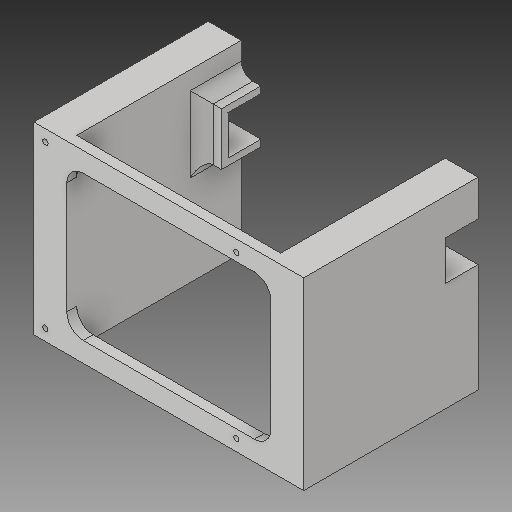
# Autodesk Inventor part: baseRaspberry
Saved by Autodesk Inventor 2018 (Build 220112000, 112)
## iProperties
Created: 2018-02-26
Part Number: baseRaspberry
Material: Genérico
Document SubType Name: Modeling
Designer: ivanb
Density: 1 g/cm^3
Appearance: Valor por defecto
Author: ivanb
Autodesk Inventor part; units mm, degrees
ref_plane "YZ Plane" through (0, 0, 0) normal (1, 0, 0) x (0, 1, 0)
ref_plane "XZ Plane" through (0, 0, 0) normal (0, 1, 0) x (-1, 0, 0)
ref_plane "XY Plane" through (0, 0, 0) normal (0, 0, 1) x (1, 0, 0)
ref_plane "Plano de trabajo1" through (-77.1004, 28.9483, 0) normal (0, 0, -1) x (-1, 0, 0)
sketch "Boceto1" plane through (-77.1004, 28.9483, 0) normal (0, 0, -1) x (-1, 0, 0)
  line L0 (82, -56) -> (-3, -56)
  line L1 (-3, -56) -> (-3, 0)
  line L2 (-3, 0) -> (82, 0)
  line L3 (82, 0) -> (82, -56)
  point P0 (-77.1004, -28.9483)
  constraints: 8 end point, 2 parallel, 1 horizontal, 1 perpendicular
extrude "Extrusión1" add sketch "Boceto1" along normal blind 20
ref_plane "Plano de trabajo3" through (-77.1004, 28.9483, 0) normal (0, 0, 1) x (1, 0, 0)
sketch "Boceto2" plane through (-77.1004, 28.9483, 0) normal (0, 0, 1) x (1, 0, 0)
  circle A0 centre (-78.5, -3.5) radius 1.375 projected
  circle A1 centre (-78.5, -3.5) radius 1.125
  circle A2 centre (-20.5, -3.5) radius 1.375 projected
  circle A3 centre (-20.5, -3.5) radius 1.125
  circle A4 centre (-20.5, -52.5) radius 1.375 projected
  circle A5 centre (-20.5, -52.5) radius 1.125
  circle A6 centre (-78.5, -52.5) radius 1.375 projected
  circle A7 centre (-78.5, -52.5) radius 1.125
  line L0 (-91.1268, 5.8368) -> (25.5851, 5.8368)
  line L1 (25.5851, 5.8368) -> (25.5851, -70.6743)
  line L2 (25.5851, -70.6743) -> (-91.1268, -70.6743)
  line L3 (-91.1268, -70.6743) -> (-91.1268, 5.8368)
  point P0 (77.1004, -28.9483)
  dimension "d3" = 2.25
  dimension "d4" = 2.25
  dimension "d5" = 2.25
  dimension "d6" = 2.25
  constraints: 8 end point, 4 centre point, 4 coincident, 2 parallel, 1 horizontal, 1 perpendicular
  measures "d3" diameter of A1
  measures "d4" diameter of A3
  measures "d5" diameter of A5
  measures "d6" diameter of A7
extrude "Extrusión2" cut sketch "Boceto2" against normal blind 10 contours L0 L1 L2 L3
ref_plane "Plano de trabajo2" through (-77.1004, 28.9483, -20) normal (0, 0, -1) x (-1, 0, 0)
sketch "Boceto8" plane through (-77.1004, 28.9483, -20) normal (0, 0, -1) x (-1, 0, 0)
  circle A0 centre (77, -31) radius 1.25
  circle A1 centre (77, -3) radius 1.25
  line L0 (-3, -56) -> (82, -56) projected
  circle A2 centre (5, -31) radius 1.25
  circle A3 centre (5, -3) radius 1.25
  line L1 (82, -56) -> (82, 0) projected
  line L2 (82, -56) -> (72, -56)
  line L3 (72, -56) -> (72, 0)
  line L4 (72, 0) -> (82, 0)
  line L5 (82, 0) -> (82, -56)
  line L6 (10.1328, -56) -> (0.1328, -56)
  line L7 (5, -31) -> (5, -3)
  line L8 (0, -52.0097) -> (0, -25.6767)
  line L9 (79, -56) -> (0, -56) projected
  line L10 (0, -56) -> (10, -56)
  line L11 (10, -56) -> (10, 0)
  line L12 (10, 0) -> (0, 0)
  line L13 (0, 0) -> (0, -56)
  line L14 (82, 0) -> (-3, 0) projected
  point P0 (-77.1004, -28.9483)
  dimension "d31" = 2.5
  dimension "d32" = 2.5
  dimension "d33" = 28
  dimension "d35" = 2.5
  dimension "d36" = 72
  dimension "d37" = 2.5
  dimension "d38" = 5
  dimension "d39" = 72
  dimension "d40" = 5
  dimension "d41" = 28
  dimension "d43" = 10
  dimension "d45" = 5
  dimension "d46" = 10
  dimension "d92" = 0
  dimension "d175" = 3
  dimension "d176" = 3
  constraints: 22 end point, 4 centre point, 4 parallel, 3 horizontal, 2 perpendicular, 1 point on line, 1 vertical
  measures "d31" diameter of A0
  measures "d32" diameter of A1
  measures "d33" distance of A1.centre A0.centre
  measures "d35" diameter of A2
  measures "d36" distance of L7.start A0.centre
  measures "d37" diameter of A3
  measures "d38" distance from line of L1 A0.centre
  measures "d39" distance of L7.end A1.centre
  measures "d40" distance from line of L1 A1.centre
  measures "d41" distance of L7.end L7.start
  measures "d43" distance of L3.end L4.end
  measures "d45" distance from line of L7.start L8
  measures "d46" distance of L12.end L11.end
  measures "d92" distance between parallel lines of L14 L12
  measures "d175" distance from line of L14 L7.end
  measures "d176" distance from line of L14 A1.centre
extrude "Extrusión8" add sketch "Boceto8" along normal blind 30 contours L13 L8 L12 L11 L0 | L3 L4 L1 L0
ref_plane "Plano de trabajo6" through (-159.1004, -27.0517, -10) normal (-1, 0, 0) x (0, 0, 1)
sketch "Boceto9" plane through (-159.1004, -27.0517, -10) normal (-1, 0, 0) x (0, 0, 1)
  line L0 (-30, 33) -> (-40, 33)
  line L1 (-40, 33) -> (-40, 45)
  line L2 (-40, 45) -> (-30, 45)
  line L3 (-30, 45) -> (-30, 33)
  line L4 (0, 0) -> (-40, 0) projected
  line L5 (-40, 0) -> (-40, 56) projected
  line L6 (0, 56) -> (-40, 56) projected
  point P0 (10, 27.0517)
  dimension "d49" = 10
  dimension "d50" = 12
  dimension "d52" = 0
  dimension "d82" = 11
  constraints: 8 end point, 2 parallel, 1 horizontal, 1 perpendicular
  measures "d49" distance of L1.end L2.end
  measures "d50" distance of L0.end L1.end
  measures "d52" distance between parallel lines of L5 L1
  measures "d82" distance between parallel lines of L6 L2
extrude "Extrusión9" cut sketch "Boceto9" against normal blind 100
ref_plane "Plano de trabajo5" through (-149.1004, -27.0517, -20) normal (1, 0, 0) x (0, 0, -1)
sketch "Boceto10" plane through (-149.1004, -27.0517, -20) normal (1, 0, 0) x (0, 0, -1)
  line L0 (18, 31) -> (30, 31)
  line L1 (30, 31) -> (30, 47)
  line L2 (30, 47) -> (18, 47)
  line L3 (18, 47) -> (18, 31)
  line L4 (-10, 56) -> (30, 56) projected
  line L5 (30, 33) -> (30, 0) projected
  line L6 (20, 33) -> (20, 45) projected
  line L7 (30, 33) -> (20, 33)
  line L8 (20, 33) -> (20, 45)
  line L9 (20, 45) -> (30, 45) projected
  line L10 (20, 45) -> (30, 45)
  point P0 (-20, 27.0517)
  dimension "d59" = 12
  dimension "d60" = 16
  dimension "d133" = 2
  constraints: 14 end point, 4 equal length, 2 perpendicular, 1 horizontal
  measures "d59" distance of L0.start L0.end
  measures "d60" distance of L0.end L1.end
  measures "d133" distance between parallel lines of L9 L2
extrude "Extrusión10" add sketch "Boceto10" along normal blind 6 contours L3 L2 L1 L9 L6 L7 L0
sketch "Boceto11" plane through (-77.1004, -27.0517, -20) normal (1, 0, 0) x (0, 0, -1)
  line L0 (30, 45) -> (30, 76)
  line L1 (18, 31) -> (30, 31)
  line L2 (30, 31) -> (30, 47)
  line L3 (30, 47) -> (18, 47)
  line L4 (18, 47) -> (18, 31)
  line L5 (30, 33) -> (20, 33)
  line L6 (20, 33) -> (30, 33)
  line L7 (30, 33) -> (20, 33)
  line L8 (20, 33) -> (20, 45)
  line L9 (20, 33) -> (20, 45)
  line L10 (30, 45) -> (20, 45)
  line L11 (20, 45) -> (30, 45)
  line L12 (20, 45) -> (30, 45) projected
  point P0 (-20, 27.0517)
  point P1 (-20, 27.0517)
  dimension "d64" = 12
  dimension "d65" = 16
  dimension "d66" = 2
  dimension "d88" = 0
  dimension "d89" = 2
  dimension "d177" = 10
  constraints: 24 end point, 3 equal length, 3 perpendicular, 1 horizontal, 1 point on line
  measures "d64" distance of L1.start L1.end
  measures "d65" distance of L1.end L2.end
  measures "d66" distance between parallel lines of L1 L5
  measures "d88" distance between parallel lines of L12 L10
  measures "d89" distance between parallel lines of L3 L10
  measures "d177" distance of L0.start L8.end
extrude "Extrusión11" add sketch "Boceto11" against normal blind 16 contours L10 L8 L5 L2 L1 L4 L3 L0
ref_plane "Plano de trabajo4" through (-159.1004, -27.0517, -10) normal (0, -1, 0) x (1, 0, 0)
sketch "Boceto12" plane through (-159.1004, -27.0517, -10) normal (0, -1, 0) x (1, 0, 0)
  line L0 (0, 0) -> (0, -40) projected
  line L1 (0, -7) -> (97.2238, -7)
  line L2 (97.2238, -7) -> (97.2238, 2.4478)
  line L3 (97.2238, 2.4478) -> (0, 2.4478)
  line L4 (0, 2.4478) -> (0, -7)
  line L5 (72, -10) -> (10, -10) projected
  point P0 (159.1004, 10)
  dimension "d69" = 3
  constraints: 8 end point, 2 parallel, 1 horizontal, 1 perpendicular, 1 point on line
  measures "d69" distance between parallel lines of L1 L5
extrude "Extrusión12" cut sketch "Boceto12" against normal blind 60
sketch "Boceto13" plane through (-155.6004, 25.4483, 0) normal (0, 0, 1) x (1, 0, 0)
  line L0 (90.0679, 13.1573) -> (-12.4886, 13.1573)
  line L1 (-12.4886, 13.1573) -> (-12.4886, -64.4116)
  line L2 (-12.4886, -64.4116) -> (90.0679, -64.4116)
  line L3 (90.0679, -64.4116) -> (90.0679, 13.1573)
  point P0 (155.6004, -25.4483)
  constraints: 8 end point, 2 parallel, 1 horizontal, 1 perpendicular
extrude "Extrusión13" cut sketch "Boceto13" against normal blind 10
ref_plane "Plano de trabajo8" through (-159.1004, -27.0517, -17) normal (0, 0, 1) x (1, 0, 0)
sketch "Boceto14" plane through (-159.1004, -27.0517, -17) normal (0, 0, 1) x (1, 0, 0)
  circle A0 centre (61.5, 52.5) radius 1
  circle A1 centre (61.5, 52.5) radius 1.375
  circle A2 centre (61.5, 3.5) radius 1
  circle A3 centre (61.5, 3.5) radius 1.375
  circle A4 centre (3.5, 3.5) radius 1
  circle A5 centre (3.5, 3.5) radius 1.375
  circle A6 centre (3.5, 52.5) radius 1
  circle A7 centre (3.5, 52.5) radius 1.375
  point P0 (159.1004, 27.0517)
  dimension "d140" = 2
  dimension "d141" = 49
  dimension "d142" = 58
  dimension "d143" = 58
  dimension "d144" = 49
  dimension "d145" = 2
  dimension "d146" = 2
  dimension "d147" = 2
  constraints: 8 centre point, 4 coincident
  measures "d140" diameter of A2
  measures "d141" distance of A1.centre A3.centre
  measures "d142" distance of A1.centre A7.centre
  measures "d143" distance of A5.centre A3.centre
  measures "d144" distance of A7.centre A5.centre
  measures "d145" diameter of A4
  measures "d146" diameter of A6
  measures "d147" diameter of A0
extrude "Extrusión14" cut sketch "Boceto14" against normal blind 10 contours A0 | A2 | A4 | A6
ref_plane "Plano de trabajo7" through (-159.1004, -27.0517, -17) normal (0, 0, 1) x (1, 0, 0)
sketch "Boceto15" plane through (-159.1004, -27.0517, -17) normal (0, 0, 1) x (1, 0, 0)
  circle A0 centre (61.5, 52.5) radius 1.375 projected
  circle A1 centre (61.5, 52.5) radius 2.5
  circle A2 centre (61.5, 3.5) radius 1.375 projected
  circle A3 centre (61.5, 3.5) radius 2.5
  circle A4 centre (3.5, 3.5) radius 1.375 projected
  circle A5 centre (3.5, 3.5) radius 2.5
  circle A6 centre (3.5, 52.5) radius 1.375 projected
  circle A7 centre (3.5, 52.5) radius 2.5
  point P0 (159.1004, 27.0517)
  dimension "d76" = 5
  dimension "d77" = 5
  dimension "d78" = 5
  dimension "d79" = 5
  constraints: 4 centre point, 4 coincident
  measures "d76" diameter of A1
  measures "d77" diameter of A3
  measures "d78" diameter of A5
  measures "d79" diameter of A7
extrude "Extrusión15" add sketch "Boceto15" along normal blind 3
sketch "Boceto16" plane through (-149.1004, -27.0517, -20) normal (0, -1, 0) x (1, 0, 0)
  line L0 (-10, 3) -> (-10, -30) projected
  line L1 (-10, 3) -> (-37, 3)
  line L2 (-37, 3) -> (-37, 0)
  line L3 (-37, 0) -> (-10, 0)
  line L4 (-10, 0) -> (-10, 3)
  point P0 (149.1004, 20)
  dimension "d93" = 27
  dimension "d94" = 3
  constraints: 8 end point, 2 parallel, 1 horizontal, 1 perpendicular
  measures "d93" distance of L3.end L2.end
  measures "d94" distance of L2.end L1.end
extrude "Extrusión16" add sketch "Boceto16" against normal blind 67
sketch "Boceto17" plane through (-74.1004, -27.0517, -17) normal (0, 0, 1) x (1, 0, 0)
  line L0 (-85.9191, 66.0479) -> (-111.9991, 66.0479)
  line L1 (-111.9991, 66.0479) -> (-111.9991, 4.6279)
  line L2 (-111.9991, 4.6279) -> (-85.9191, 4.6279)
  line L3 (-85.9191, 4.6279) -> (-85.9191, 66.0479)
  line L4 (-91.7766, 35.3379) -> (-98.9591, 35.3379)
  line L5 (-98.9591, 35.3379) -> (-98.9591, 28.1123)
  circle A0 centre (-88.4591, 63.5879) radius 1
  circle A1 centre (-88.4591, 7.0879) radius 1
  circle A2 centre (-109.4591, 63.5879) radius 1
  circle A3 centre (-109.4591, 7.0879) radius 1
  point P0 (74.1004, 27.0517)
  dimension "d97" = 26.08
  dimension "d98" = 61.42
  dimension "d99" = 2
  dimension "d100" = 28.25
  dimension "d101" = 10.5
  constraints: 12 end point, 4 centre point, 3 symmetric about line, 2 horizontal, 2 parallel, 1 perpendicular, 1 vertical, 5 other
  measures "d97" distance of L1.end L2.end
  measures "d98" distance of L0.end L1.end
  measures "d99" diameter of A0
  measures "d100" distance from line of L4 A0.centre
  measures "d101" distance from line of A0.centre L5
extrude "Extrusión17" cut sketch "Boceto17" against normal blind 56 contours A0 | A1 | A2 | A3
sketch "Boceto18" plane through (-74.1004, -27.0517, -17) normal (0, 0, 1) x (1, 0, 0)
  circle A0 centre (-109.4591, 63.5879) radius 1 projected
  circle A1 centre (-88.4591, 63.5879) radius 1 projected
  circle A2 centre (-88.4591, 7.0879) radius 1 projected
  circle A3 centre (-109.4591, 7.0879) radius 1 projected
  circle A4 centre (-81.5, 3.5) radius 2.5 projected
  circle A5 centre (-23.5, 52.5) radius 2.5 projected
  circle A6 centre (-23.5, 3.5) radius 2.5 projected
  circle A7 centre (-81.5, 52.5) radius 2.5 projected
  line L0 (0, 56) -> (0, 0) projected
  line L1 (-85, 56) -> (0, 56) projected
  line L2 (-85, 56) -> (-85, 67) projected
  line L3 (-112, 67) -> (-85, 67) projected
  line L4 (-112, 0) -> (-112, 67) projected
  line L5 (0, 0) -> (-112, 0) projected
  circle A8 centre (-88.4591, 63.5879) radius 2.25
  circle A9 centre (-109.4591, 63.5879) radius 2.25
  circle A10 centre (-88.4591, 7.0879) radius 2.25
  circle A11 centre (-109.4591, 7.0879) radius 2.25
  point P0 (74.1004, 27.0517)
  dimension "d104" = 5
  dimension "d105" = 4.5
  dimension "d106" = 4.5
  dimension "d107" = 4.5
  dimension "d108" = 4.5
  constraints: 4 centre point, 4 coincident
  measures "d104" diameter of A7
  measures "d105" diameter of A8
  measures "d106" diameter of A9
  measures "d107" diameter of A10
  measures "d108" diameter of A11
extrude "Extrusión18" add sketch "Boceto18" along normal blind 3 contours A8 | A9 | A10 | A11
fillet "Empalme1" radius 4 1 edges at (-186.1004, -27.0517, -18.5)
sketch "Boceto19" plane through (-74.1004, -27.0517, -17) normal (0, 0, 1) x (1, 0, 0)
  line L0 (-85, 0) -> (-85, 33) projected
  line L1 (-85, 4.1487) -> (-113.131, 4.1487)
  line L2 (-113.131, 4.1487) -> (-113.131, -0.5367)
  line L3 (-113.131, -0.5367) -> (-85, -0.5367)
  line L4 (-85, -0.5367) -> (-85, 4.1487)
  point P0 (74.1004, 27.0517)
  constraints: 8 end point, 2 parallel, 1 horizontal, 1 perpendicular, 1 point on line
extrude "Extrusión19" cut sketch "Boceto19" against normal blind 3
fillet "Empalme2" radius 4 1 edges at (-186.1004, -22.903, -18.5)
fillet "Empalme3" radius 3 2 edges at (-159.1004, 39.9483, -18.5) (-186.1004, 39.9483, -18.5)
sketch "Boceto30" plane through (-149.1004, -27.0517, -20) normal (1, 0, 0) x (0, 0, -1)
  line L0 (18, 31) -> (18, 47) projected
  line L1 (0, 0) -> (0, 56) projected
  line L2 (18, 30.6682) -> (0, 30.6682)
  line L3 (0, 30.6682) -> (0, 33.6682)
  line L4 (0, 33.6682) -> (18, 33.6682)
  line L5 (18, 33.6682) -> (18, 30.6682)
  line L6 (0, 0) -> (30, 0) projected
  line L7 (0, 0) -> (3, 0)
  line L8 (3, 0) -> (3, 30.6682)
  line L9 (3, 30.6682) -> (0, 30.6682)
  line L10 (0, 30.6682) -> (0, 0)
  point P0 (-20, 27.0517)
  dimension "d180" = 3
  dimension "d181" = 3
  constraints: 16 end point, 4 parallel, 3 point on line, 2 horizontal, 2 perpendicular
  measures "d180" distance of L2.end L3.end
  measures "d181" distance of L9.end L8.end
extrude "Extrusión28" [suppressed]
sketch "Boceto31" plane through (-149.1004, -27.0517, -50) normal (1, 0, 0) x (0, 0, -1)
  line L0 (-30, 0) -> (0, 0) projected
  line L1 (-27, 0) -> (-30, 0)
  line L2 (-30, 0) -> (-30, 30.6387)
  line L3 (-30, 30.6387) -> (-27, 30.6387)
  line L4 (-27, 30.6387) -> (-27, 0)
  line L5 (-30, 33.6682) -> (-12, 33.6682) projected
  line L6 (-27, 30.6682) -> (-15.8407, 30.6682)
  line L7 (-15.8407, 30.6682) -> (-15.8407, 33.6682)
  line L8 (-15.8407, 33.6682) -> (-27, 33.6682)
  line L9 (-27, 33.6682) -> (-27, 30.6682)
  point P0 (-50, 27.0517)
  constraints: 16 end point, 4 parallel, 2 horizontal, 2 perpendicular, 1 point on line
sketch "Boceto33" plane through (-77.1004, 28.9483, -50) normal (0, 0, -1) x (-1, 0, 0)
  line L0 (82, -23) -> (66, -23) projected
  line L1 (66, -25) -> (66, -23) projected
  line L2 (72, -25) -> (66, -25) projected
  line L3 (72, -25) -> (72, -56) projected
  line L4 (72, -56) -> (82, -56) projected
  circle A0 centre (77, -31) radius 1.25 projected
  circle A1 centre (77, -3) radius 1.25 projected
  line L5 (66, -11) -> (82, -11) projected
  line L6 (72, 0) -> (72, -9) projected
  line L7 (72, -9) -> (66, -9) projected
  line L8 (66, -11) -> (66, -9) projected
  line L9 (10, -9) -> (10, 0) projected
  line L10 (10, 0) -> (0, 0) projected
  line L11 (0, 0) -> (0, -11) projected
  line L12 (0, -11) -> (16, -11) projected
  line L13 (16, -9) -> (16, -11) projected
  line L14 (10, -9) -> (16, -9) projected
  circle A2 centre (5, -31) radius 1.25 projected
  line L15 (0, -23) -> (0, -56) projected
  line L16 (0, -56) -> (10, -56) projected
  line L17 (10, -56) -> (10, -25) projected
  line L18 (10, -25) -> (16, -25) projected
  line L19 (16, -23) -> (16, -25) projected
  line L20 (0, -23) -> (16, -23) projected
  line L21 (10, -9) -> (10, 0) projected
  line L22 (10, 0) -> (0, 0) projected
  line L23 (0, 0) -> (0, -11) projected
  line L24 (0, -11) -> (16, -11) projected
  line L25 (16, -9) -> (16, -11) projected
  line L26 (10, -9) -> (16, -9) projected
  line L27 (82, -11) -> (82, 0) projected
  line L28 (82, 0) -> (72, 0) projected
  line L29 (82, -56) -> (82, -23) projected
  circle A3 centre (5, -3) radius 1.25 projected
  point P0 (-77.1004, -28.9483)
extrude "Extrusión29" add sketch "Boceto33" along normal blind 20
sketch "Boceto34" plane through (-149.1004, 3.9483, -38) normal (0, -1, 0) x (1, 0, 0)
  line L0 (6, -32) -> (0, -32)
  line L1 (0, -32) -> (0, -22)
  line L2 (0, -22) -> (6, -22)
  line L3 (6, -22) -> (6, -32)
  line L4 (0, 18) -> (0, -32) projected
  line L5 (6, -22) -> (0, -22)
  line L6 (0, -22) -> (0, 1.0626)
  line L7 (0, 1.0626) -> (6, 1.0626)
  line L8 (6, 1.0626) -> (6, -22)
  line L9 (56, 0) -> (56, -32) projected
  line L10 (62, 0) -> (62, -32) projected
  line L11 (56, -32) -> (62, -32)
  line L12 (62, -32) -> (62, -22)
  line L13 (62, -22) -> (56, -22)
  line L14 (56, -22) -> (56, -32)
  line L15 (62, 0) -> (56, 0) projected
  line L16 (62, -22) -> (56, -22)
  line L17 (56, -22) -> (56, 0)
  line L18 (56, 0) -> (62, 0)
  line L19 (62, 0) -> (62, -22)
  point P0 (149.1004, 38)
  point P1 (0, 15)
  point P2 (0, -12)
  point P3 (56, -12)
  point P4 (62, -12)
  dimension "d188" = 6
  dimension "d189" = 10
  dimension "d190" = 10
  constraints: 32 end point, 8 parallel, 4 horizontal, 4 perpendicular, 2 point on line
  measures "d188" distance of L1.end L2.end
  measures "d189" distance of L0.end L1.end
  measures "d190" distance of L12.end L11.end
extrude "Extrusión30" cut sketch "Boceto34" against normal blind 20 contours L2 L4 L7 L8 | L15 L10 L13 L9
sketch "Boceto35" plane through (-149.1004, 3.9483, -70) normal (0, -1, 0) x (1, 0, 0)
  line L0 (6, 10) -> (0, 10)
  line L1 (0, 10) -> (0, 12)
  line L2 (0, 12) -> (6, 12)
  line L3 (6, 12) -> (6, 10)
  line L4 (56, 10) -> (56, 0) projected
  line L5 (62, 50) -> (62, 0) projected
  line L6 (56, 10) -> (62, 10)
  line L7 (62, 10) -> (62, 12)
  line L8 (62, 12) -> (56, 12)
  line L9 (56, 12) -> (56, 10)
  line L10 (0, 10) -> (6, 10) projected
  line L11 (-10, 30) -> (0, 30) projected
  line L12 (0, 10) -> (-10, 10)
  line L13 (-10, 10) -> (-10, 30)
  line L14 (-10, 30) -> (0, 30)
  line L15 (0, 30) -> (0, 10)
  line L16 (62, 10) -> (62, 30) projected
  line L17 (72, 0) -> (72, 30) projected
  line L18 (62, 10) -> (72, 10)
  line L19 (72, 10) -> (72, 30)
  line L20 (72, 30) -> (62, 30)
  line L21 (62, 30) -> (62, 10)
  point P0 (149.1004, 70)
  point P1 (62, 47)
  dimension "d193" = 6
  dimension "d194" = 2
  constraints: 32 end point, 8 parallel, 4 horizontal, 4 perpendicular, 2 point on line
  measures "d193" distance of L1.end L2.end
  measures "d194" distance of L0.end L1.end
extrude "Extrusión31" add sketch "Boceto35" against normal blind 16
sketch "Boceto36" plane through (-149.1004, -27.0517, -23) normal (1, 0, 0) x (0, 0, -1)
  line L0 (-3, 56) -> (47, 56) projected
  line L1 (-3, 0) -> (-3, 56) projected
  line L2 (-3, 0) -> (47, 0) projected
  line L3 (15, 30.6682) -> (15, 33.6682) projected
  line L4 (35, 24) -> (35, 40) projected
  line L5 (15, 30.6682) -> (35, 30.6682)
  line L6 (35, 30.6682) -> (35, 33.6682)
  line L7 (35, 33.6682) -> (15, 33.6682)
  line L8 (15, 33.6682) -> (15, 30.6682)
  line L9 (35, 47) -> (47, 47) projected
  line L10 (47, 31) -> (47, 0) projected
  line L11 (47, 31) -> (35, 31) projected
  line L12 (35, 31) -> (35, 47) projected
  line L13 (47, 56) -> (47, 47) projected
  point P0 (-23, 27.0517)
  constraints: 8 end point, 2 parallel, 1 horizontal, 1 perpendicular, 1 point on line
extrude "Extrusión32" [suppressed]
sketch "Boceto37" plane through (-159.1004, -27.0517, -17) normal (0, 0, 1) x (1, 0, 0)
  circle A0 centre (5, 25) radius 1.25 projected
  line L0 (0, 33) -> (16, 33) projected
  line L1 (16, 33) -> (16, 31) projected
  line L2 (16, 31) -> (10, 31) projected
  line L3 (10, 31) -> (10, 0) projected
  line L4 (10, 0) -> (0, 0) projected
  circle A1 centre (5, 53) radius 1.25 projected
  line L5 (72, 47) -> (72, 56) projected
  line L6 (72, 56) -> (82, 56) projected
  line L7 (82, 56) -> (82, 45) projected
  line L8 (82, 45) -> (66, 45) projected
  line L9 (66, 45) -> (66, 47) projected
  line L10 (66, 47) -> (72, 47) projected
  circle A2 centre (77, 25) radius 1.25 projected
  line L11 (82, 33) -> (82, 0) projected
  line L12 (82, 0) -> (72, 0) projected
  line L13 (72, 0) -> (72, 31) projected
  line L14 (72, 31) -> (66, 31) projected
  line L15 (66, 31) -> (66, 33) projected
  line L16 (66, 33) -> (82, 33) projected
  line L17 (66, 33) -> (82, 33) projected
  line L18 (66, 33) -> (66, 45) projected
  line L19 (82, 45) -> (66, 45) projected
  line L20 (82, 33) -> (82, 45) projected
  line L21 (16, 33) -> (16, 45) projected
  line L22 (0, 33) -> (16, 33) projected
  line L23 (0, 33) -> (0, 45) projected
  line L24 (10, 50.0297) -> (72, 50.0297)
  line L25 (72, 50.0297) -> (72, 6.0297)
  line L26 (72, 6.0297) -> (10, 6.0297)
  line L27 (10, 6.0297) -> (10, 50.0297)
  line L28 (0, 0) -> (0, 33) projected
  line L29 (16, 45) -> (0, 45) projected
  point P0 (159.1004, 27.0517)
  dimension "d201" = 44
  dimension "d202" = 62
  dimension "d203" = 0
  constraints: 8 end point, 2 parallel, 1 horizontal, 1 perpendicular
  measures "d201" distance of L24.end L25.end
  measures "d202" distance of L24.start L24.end
  measures "d203" distance between parallel lines of L5 L25
extrude "Extrusión33" cut sketch "Boceto37" against normal blind 10 contours L27 L29 L21 L0 | L0 L1 L2 L27 | L21 L29 L27 L24 L5 L10 L9 L18 L15 L14 L13 L26 L3 L2 L1 | L14 L15 L16 L25 | L25 L8 L9 L10 | L16 L18 L8 L25
sketch "Boceto38" plane through (-159.1004, -27.0517, -17) normal (0, 0, 1) x (1, 0, 0)
  line L0 (-22.2573, 61.4882) -> (-6.2573, 61.4882)
  line L1 (-6.2573, 61.4882) -> (-6.2573, 9.4882)
  line L2 (-6.2573, 9.4882) -> (-22.2573, 9.4882)
  line L3 (-22.2573, 9.4882) -> (-22.2573, 61.4882)
  point P0 (159.1004, 27.0517)
  dimension "d206" = 16
  dimension "d207" = 52
  constraints: 8 end point, 2 parallel, 1 horizontal, 1 perpendicular
  measures "d206" distance of L1.end L2.end
  measures "d207" distance of L0.end L1.end
extrude "Extrusión34" cut sketch "Boceto38" against normal blind 10
fillet "Empalme4" radius 5 4 edges at (-181.3578, 34.4365, -18.5) (-165.3578, 34.4365, -18.5) (-165.3578, -17.5635, -18.5) (-181.3578, -17.5635, -18.5)
fillet "Empalme5" radius 5 4 edges at (-149.1004, 22.9781, -18.5) (-87.1004, 22.9781, -18.5) (-149.1004, -21.0219, -18.5) (-87.1004, -21.0219, -18.5)
sketch "Boceto39" plane through (-159.1004, -22.903, -20) normal (-1, 0, 0) x (0, 0, 1)
  circle A0 centre (44.0116, 14.0123) radius 1.0922 projected
  circle A1 centre (30.5496, -1.9897) radius 1.0922 projected
  point P0 (20, 22.903)
extrude "Extrusión35" cut sketch "Boceto39" against normal blind 5
sketch "Boceto40" plane through (-159.1004, -27.0517, -17) normal (0, 0, 1) x (1, 0, 0)
  line L0 (-22.2573, 14.4882) -> (-22.2573, 56.4882) projected
  arc A0 (-17.2573, 61.4882) -> (-22.2573, 56.4882) centre (-17.2573, 56.4882) ccw projected
  line L1 (-17.2573, 61.4882) -> (-11.2573, 61.4882) projected
  arc A1 (-6.2573, 56.4882) -> (-11.2573, 61.4882) centre (-11.2573, 56.4882) ccw projected
  line L2 (-6.2573, 56.4882) -> (-6.2573, 14.4882) projected
  arc A2 (-11.2573, 9.4882) -> (-6.2573, 14.4882) centre (-11.2573, 14.4882) ccw projected
  line L3 (-11.2573, 9.4882) -> (-17.2573, 9.4882) projected
  arc A3 (-22.2573, 14.4882) -> (-17.2573, 9.4882) centre (-17.2573, 14.4882) ccw projected
  circle A4 centre (3.5, 52.5) radius 2.5 projected
  circle A5 centre (61.5, 3.5) radius 2.5 projected
  line L4 (61.8845, 50.0297) -> (67, 50.0297) projected
  arc A6 (72, 45.0297) -> (67, 50.0297) centre (67, 45.0297) ccw projected
  line L5 (72, 45.0297) -> (72, 11.0297) projected
  arc A7 (67, 6.0297) -> (72, 11.0297) centre (67, 11.0297) ccw projected
  line L6 (67, 6.0297) -> (15, 6.0297) projected
  arc A8 (10, 11.0297) -> (15, 6.0297) centre (15, 11.0297) ccw projected
  line L7 (10, 11.0297) -> (10, 45.0297) projected
  arc A9 (15, 50.0297) -> (10, 45.0297) centre (15, 45.0297) ccw projected
  line L8 (15, 50.0297) -> (61.1155, 50.0297) projected
  arc A10 (61.8845, 50.0297) -> (61.1155, 50.0297) centre (61.5, 52.5) ccw projected
  circle A11 centre (3.5, 3.5) radius 2.5 projected
  circle A12 centre (-24.4591, 63.5879) radius 2.25 projected
  circle A13 centre (-3.4591, 63.5879) radius 2.25 projected
  circle A14 centre (-3.4591, 7.0879) radius 2.25 projected
  arc A15 (-24, 67) -> (-27, 64) centre (-24, 64) ccw projected
  line L9 (-27, 8.1487) -> (-27, 64) projected
  arc A16 (-27, 8.1487) -> (-26.6087, 6.4232) centre (-23, 8.1487) ccw projected
  arc A17 (-25.7545, 5.2482) -> (-26.6087, 6.4232) centre (-24.4591, 7.0879) ccw projected
  arc A18 (-25.7545, 5.2482) -> (-23, 4.1487) centre (-23, 8.1487) ccw projected
  line L10 (-23, 4.1487) -> (0, 4.1487) projected
  line L11 (0, 4.1487) -> (0, 0) projected
  line L12 (85, 0) -> (0, 0) projected
  line L13 (85, 56) -> (85, 0) projected
  line L14 (0, 56) -> (85, 56) projected
  line L15 (0, 56) -> (0, 64) projected
  arc A19 (0, 64) -> (-3, 67) centre (-3, 64) ccw projected
  line L16 (-24, 67) -> (-3, 67) projected
  line L17 (0, 45) -> (0, 56) projected
  line L18 (0, 56) -> (0, 4.1487)
  circle A20 centre (-24.4591, 7.0879) radius 1 projected
  arc A21 (-25.7545, 5.2482) -> (-26.6087, 6.4232) centre (-24.4591, 7.0879) ccw projected
  arc A22 (-26.6087, 6.4232) -> (-25.7545, 5.2482) centre (-23, 8.1487) ccw projected
  arc A23 (-25.7545, 5.2482) -> (-26.6087, 6.4232) centre (-24.4591, 7.0879) ccw projected
  circle A24 centre (-24.4591, 7.0879) radius 1 projected
  point P0 (159.1004, 27.0517)
  constraints: 2 end point, 1 collinear
extrude "Extrusión36" cut sketch "Boceto40" against normal blind 5 and the other way blind 5 contours A12 | A13 | A14 | L16 A19 L15 L17 L18 L10 A18 A17 A16 L9 A15 | A17 A22 | A20
sketch "Boceto42" plane through (-159.1004, -27.0517, -17) normal (0, -1, 0) x (1, 0, 0)
  line L0 (72, -3) -> (72, -53) projected
  line L1 (82, -3) -> (82, -53) projected
  line L2 (85, -3) -> (82, -3) projected
  line L3 (85, 0) -> (85, -3) projected
  line L4 (85, 0) -> (0, 0) projected
  line L5 (0, 0) -> (0, -53) projected
  line L6 (10, -3) -> (10, -53) projected
  line L7 (72, -3) -> (10, -3) projected
  line L8 (82, -3) -> (85, -3) projected
  line L9 (82, -3) -> (82, 0)
  line L10 (10, -53) -> (0, -53) projected
  line L11 (82, -53) -> (72, -53) projected
  point P0 (159.1004, 17)
  constraints: 2 end point, 1 perpendicular, 1 point on line
extrude "Extrusión38" cut sketch "Boceto42" against normal blind 60 contours L9 L4 L3 L2
fillet "Empalme7" radius 3.5 6 edges at (-149.1004, 11.9483, -58) (-87.1004, 11.9483, -58) (-87.1004, 3.9483, -64) (-149.1004, 3.9483, -64) (-149.1004, 19.9483, -64) (-87.1004, 19.9483, -64)
sketch "Boceto43" plane through (-159.1004, 28.9483, -17) normal (0, 0, 1) x (1, 0, 0)
  line L0 (82, -56) -> (82, 0) projected
  line L1 (0, 0) -> (82, 0) projected
  line L2 (0, 0) -> (0, -56) projected
  line L3 (82, -56) -> (0, -56) projected
  circle A0 centre (3.5, -3.5) radius 2.5 projected
  circle A1 centre (61.5, -52.5) radius 2.5 projected
  line L4 (61.8845, -5.9703) -> (67, -5.9703) projected
  arc A2 (72, -10.9703) -> (67, -5.9703) centre (67, -10.9703) ccw projected
  line L5 (72, -10.9703) -> (72, -44.9703) projected
  arc A3 (67, -49.9703) -> (72, -44.9703) centre (67, -44.9703) ccw projected
  line L6 (67, -49.9703) -> (15, -49.9703) projected
  arc A4 (10, -44.9703) -> (15, -49.9703) centre (15, -44.9703) ccw projected
  line L7 (10, -44.9703) -> (10, -10.9703) projected
  arc A5 (15, -5.9703) -> (10, -10.9703) centre (15, -10.9703) ccw projected
  line L8 (15, -5.9703) -> (61.1155, -5.9703) projected
  arc A6 (61.8845, -5.9703) -> (61.1155, -5.9703) centre (61.5, -3.5) ccw projected
  circle A7 centre (3.5, -52.5) radius 2.5 projected
  circle A8 centre (61.5, -3.5) radius 2.5 projected
  point P0 (159.1004, -28.9483)
extrude "Extrusión39" cut sketch "Boceto43" along normal blind 5 contours A0 | A1 | A8 A6 | A7
thicken "Engrosado5" operation add thickness 0.2 both sides no extend neighbours yes toward (0.0402659, -0.999189, 0) faces at (-155.6407, -22.5525, -23.6667)
thicken "Engrosado6" operation add thickness 0.2 both sides no extend neighbours yes toward (0.0402659, -0.999189, 0) faces at (-97.6407, -22.5525, -19)
thicken "Engrosado7" operation add thickness 0.2 both sides no extend neighbours yes toward (-0.354109, 0.9352042, 0) faces at (-155.2463, 24.5131, -23.6667)
thicken "Engrosado8" operation add thickness 0.2 both sides no extend neighbours yes toward (0.0402659, -0.999189, 0) faces at (-97.6407, 26.4475, -19)
sketch "Boceto44" plane through (-159.1004, -27.0517, -17) normal (-1, 0, 0) x (0, 0, 1)
  circle A0 centre (-5.0437, 19.161) radius 1.0922 projected
  circle A1 centre (-18.5057, 3.159) radius 1.0922 projected
  point P0 (17, 27.0517)
extrude "Extrusión40" cut sketch "Boceto44" against normal blind 5
thicken "Engrosado11" operation add thickness 0.2 both sides no extend neighbours yes toward (0, 0.1604113, -0.9870503) faces at (-155.7671, -8.0659, -20.9657)
thicken "Engrosado12" operation add thickness 0.2 both sides no extend neighbours yes toward (0, 0.1604113, -0.9870503) faces at (-155.7671, -24.0679, -34.4277)
